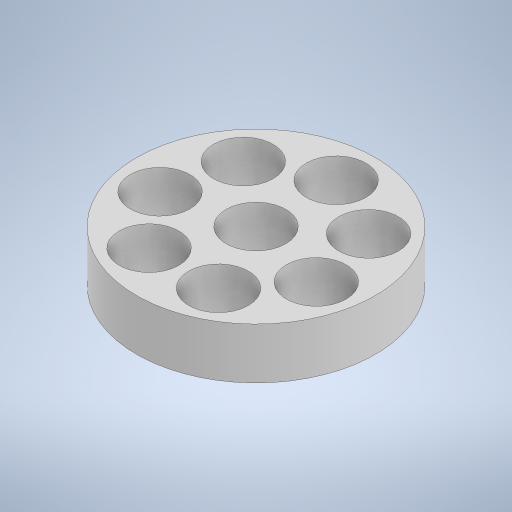
# Autodesk Inventor part: braided_terminal_end_4.1mm_8ea
Saved by Autodesk Inventor 2024 (Build 280153000, 153)
## iProperties
Created: 2024-07-10
Part Number: braided_terminal_end_4.1mm_8ea
Material: 일반
Document SubType Name: Modeling
Designer: Gihyeok Na
Density: 1 g/cm^3
Appearance: 기본값
Author: Gihyeok Na
Autodesk Inventor part; units mm, degrees
ref_plane "YZ Plane" through (0, 0, 0) normal (1, 0, 0) x (0, 1, 0)
ref_plane "XZ Plane" through (0, 0, 0) normal (0, 1, 0) x (-1, 0, 0)
ref_plane "XY Plane" through (0, 0, 0) normal (0, 0, 1) x (1, 0, 0)
sketch "스케치1" plane through (0, 0, 0) normal (0, 1, 0) x (-1, 0, 0)
  circle A0 centre (0, 0) radius 2.05
  line L0 (0, 0) -> (0, -15.8678) construction
  circle A1 centre (0, -5.5) radius 2.05
  line L1 (0, 0) -> (12.4059, -9.8934) construction
  circle A2 centre (4.3001, -3.4292) radius 2.05
  line L2 (0, 0) -> (15.4699, 3.5309) construction
  circle A3 centre (5.3621, 1.2239) radius 2.05
  line L3 (0, 0) -> (6.8848, 14.2964) construction
  circle A4 centre (2.3864, 4.9553) radius 2.05
  line L4 (0, 0) -> (-6.8848, 14.2964) construction
  circle A5 centre (-2.3864, 4.9553) radius 2.05
  line L5 (0, 0) -> (-15.4699, 3.5309) construction
  circle A6 centre (-5.3621, 1.2239) radius 2.05
  line L6 (0, 0) -> (-12.4059, -9.8934) construction
  circle A7 centre (-4.3001, -3.4292) radius 2.05
  circle A8 centre (0, 0) radius 8.2
  dimension "d0" = 4.1
  dimension "d2" = 4.1
  dimension "d3" = 5.5
  dimension "d6" = 360
  dimension "d8" = 16.4
  constraints: 14 end point, 9 centre point, 7 point on line, 2 coincident, 1 vertical, 36 other
  measures "d0" diameter of A0
  measures "d2" diameter of A1
  measures "d3" distance of A1.centre point (0, 0)
  measures "d8" diameter of A8
extrude "돌출1" add sketch "스케치1" along normal blind 3.5
